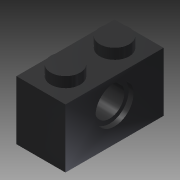
# Autodesk Inventor part: real LEGO Technic Brick 1x2 with Holes
Saved by Autodesk Inventor 2013 (Build 170138000, 138)
## iProperties
Created: 2013-06-01
Part Number: real LEGO Technic Brick 1x2 with Holes
Material: Generic
Document SubType Name: Modeling
Designer: Masta
Density: 1 g/cm^3
Author: Masta
Autodesk Inventor part; units mm, degrees
note: some values were not read from the file. Chosen so that the rebuilt part matches the saved one: arc direction of "Extrusion7".
ref_plane "YZ Plane" through (0, 0, 0) normal (1, 0, 0) x (0, 1, 0)
ref_plane "XZ Plane" through (0, 0, 0) normal (0, 1, 0) x (-1, 0, 0)
sketch "Sketch1" plane through (0, 0, 0) normal (0, 0, 1) x (1, 0, 0)
  line L0 (-4, -4) -> (4, -4)
  line L1 (4, -4) -> (4, 4)
  line L2 (4, 4) -> (-4, 4)
  line L3 (-4, 4) -> (-4, -4)
  line L4 (-4, -4) -> (4, 4) construction
  line L5 (4, -4) -> (-4, 4) construction
  circle A0 centre (0, 0) radius 2.4
  dimension "d0" = 8
  dimension "d1" = 8
  dimension "d2" = 4.8
  constraints: 12 end point, 2 midpoint, 2 parallel, 1 centre point, 1 coincident, 1 horizontal, 1 perpendicular
  measures "d0" distance of L2.end L1.end
  measures "d1" distance of L1.end L0.end
  measures "d2" diameter of A0
extrude "Extrusion1" add sketch "Sketch1" along normal blind 9.6 contours L3 L2 L1 L0 | A0
extrude "Extrusion2" add sketch "Sketch1" along normal blind 11.3 contours A0
pattern_linear "Rectangular Pattern1" count 2 spacing 8 along (0, 1, 0) of "Extrusion1", "Extrusion2"
sketch "Sketch3" plane through (0, 0, 0) normal (0, 0, -1) x (-1, 0, 0)
  line L0 (4, -4) -> (-4, -4) projected
  line L1 (4, 12) -> (4, -4) projected
  line L2 (-4, 12) -> (4, 12) projected
  line L3 (-4, -4) -> (-4, 12) projected
  line L4 (2.4, 10.4) -> (2.4, -2.4)
  line L5 (2.4, -2.4) -> (-2.4, -2.4)
  line L6 (-2.4, -2.4) -> (-2.4, 10.4)
  line L7 (-2.4, 10.4) -> (2.4, 10.4)
  circle A0 centre (0, 4) radius 1.6
  line L8 (0, -2.4) -> (0, 4) construction
  point P0 (0, 0)
  dimension "d22" = 1.6
  dimension "d23" = 3.2
  dimension "d24" = 8
  constraints: 10 end point, 1 centre point, 1 midpoint, 1 perpendicular, 3 other
  measures "d22" distance between parallel lines of L3 L6
  measures "d23" diameter of A0
  measures "d24" distance from line of L0 L8.end
extrude "Extrusion6" cut sketch "Sketch3" against normal blind 8 contours L4 L5 L6 L7
sketch "Sketch2" plane through (4, -4, 9.6) normal (1, 0, 0) x (0, 0, -1)
  circle A0 centre (4, 8) radius 2.4
  circle A1 centre (4, 8) radius 3.1
  circle A2 centre (4, 8) radius 4
  line L0 (0, 0) -> (0, 16) projected
  line L1 (4, 4) -> (0, 4)
  line L2 (4, 12) -> (0, 12)
  line L3 (9.6, 0) -> (9.6, 16) projected
  line L4 (9.6, 0) -> (0, 0) projected
  point P0 (9.6, 4)
  dimension "d12" = 4.8
  dimension "d14" = 6.2
  dimension "d29" = 8
  dimension "d30" = 8
  dimension "d31" = 5.6
  constraints: 4 end point, 3 centre point, 2 coincident, 2 perpendicular, 2 point on circle, 2 point on line, 2 tangent
  measures "d12" diameter of A0
  measures "d14" diameter of A1
  measures "d29" diameter of A2
  measures "d30" distance from line of A0.centre L4
  measures "d31" distance from line of L3 A0.centre
ref_plane "Work Plane1" through (0, -4, 9.6) normal (1, 0, 0) x (0, 0, -1)
extrude "Extrusion4" cut sketch "Sketch2" against normal up to surface (8 mm away) from surface at 0 contours A0
extrude "Extrusion5" cut sketch "Sketch2" against normal blind 0.8 contours A1
mirror "Mirror1" about plane through (0, -4, 9.6) normal (1, 0, 0) of "Extrusion5"
pattern_of_one "Rectangular Pattern2"
extrude "Extrusion7" add sketch "Sketch2" against normal up to surface (4.8 mm away) from surface at -1.6 contours A1 | A2 | A2 L0 L2 | L1 L0 A2
equation "\"d11\" = d0"
equation "\"d21\" = d0"
body "Solid1"
